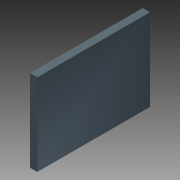
# Autodesk Inventor part: Lead Box Cover
Saved by Autodesk Inventor 2015 SP1 (Build 190203100, 203)
## iProperties
Created: 2015-03-04
Part Number: Lead Box Cover
Material: Lead
Document SubType Name: Modeling
Designer: Andrew
Density: 11.34 g/cm^3
Appearance: Lead
Author: Andrew
Autodesk Inventor part; units mm, degrees
ref_plane "YZ Plane" through (0, 0, 0) normal (1, 0, 0) x (0, 1, 0)
ref_plane "XZ Plane" through (0, 0, 0) normal (0, 1, 0) x (-1, 0, 0)
ref_plane "XY Plane" through (0, 0, 0) normal (0, 0, 1) x (1, 0, 0)
sketch "Sketch1" plane through (0, 0, 0) normal (1, 0, 0) x (0, 1, 0)
  line L0 (-24.5875, 17.8815) -> (24.5875, 17.8815)
  line L1 (24.5875, 17.8815) -> (24.5875, -17.8815)
  line L2 (24.5875, -17.8815) -> (-24.5875, -17.8815)
  line L3 (-24.5875, -17.8815) -> (-24.5875, 17.8815)
  line L4 (-24.5875, 17.8815) -> (24.5875, -17.8815) construction
  line L5 (24.5875, 17.8815) -> (-24.5875, -17.8815) construction
  point P0 (0, 0)
  dimension "d0" = 49.175
  dimension "d1" = 35.763
  constraints: 12 end point, 2 midpoint, 2 parallel, 1 horizontal, 1 perpendicular
  measures "d0" distance between parallel lines of L3 L1
  measures "d1" distance between parallel lines of L2 L0
extrude "Extrusion1" add sketch "Sketch1" along normal blind 3.175
body "Solid1"
